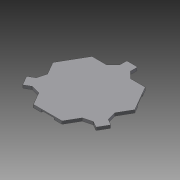
# Autodesk Inventor part: Frame_Bed
Saved by Autodesk Inventor 2014 (Build 180170000, 170)
## iProperties
Created: 2014-08-27
Part Number: Frame_Bed
Material: Generic
Document SubType Name: Modeling
Designer: ThatOtherGuy
Density: 1 g/cm^3
Appearance: Default
Author: ThatOtherGuy
Autodesk Inventor part; units mm, degrees
ref_plane "YZ Plane" through (0, 0, 0) normal (1, 0, 0) x (0, 1, 0)
ref_plane "XZ Plane" through (0, 0, 0) normal (0, 1, 0) x (-1, 0, 0)
ref_plane "XY Plane" through (0, 0, 0) normal (0, 0, 1) x (1, 0, 0)
sketch "Sketch2" plane through (0, 0, 0) normal (0, 0, 1) x (1, 0, 0)
  line L0 (0, 0) -> (-63.75, 36.8061)
  line L1 (63.75, 36.8061) -> (0, 0)
  line L2 (0, 0) -> (147.7389, 0) construction
  line L3 (63.75, 36.8061) -> (42.5, 73.6122)
  line L4 (-42.5, 73.6122) -> (-63.75, 36.8061)
  line L5 (-42.5, 73.6122) -> (42.5, 73.6122)
  line L6 (-12.5, 73.6122) -> (-12.5, 105)
  line L7 (12.5, 105) -> (12.5, 73.6122)
  line L8 (63.75, 36.8061) -> (85, 0) construction
  line L9 (12.5, 88.6122) -> (27.5, 73.6122)
  line L10 (-27.5, 73.6122) -> (-12.5, 88.6122)
  line L11 (63.75, 36.8061) -> (77.9423, 45)
  line L12 (77.9423, 45) -> (61.423, 73.6122)
  line L13 (61.423, 73.6122) -> (42.5, 73.6122)
  line L14 (-63.75, 36.8061) -> (-77.9423, 45)
  line L15 (-77.9423, 45) -> (-61.423, 73.6122)
  line L16 (-61.423, 73.6122) -> (-42.5, 73.6122)
  line L17 (-12.5, 105) -> (12.5, 105)
  dimension "d29" = 120
  dimension "d30" = 30
  dimension "d31" = 30
  dimension "d33" = 25
  dimension "d34" = 85
  dimension "d35" = 60
  dimension "d36" = 85
  dimension "d37" = 45
  dimension "d38" = 15
  dimension "d45" = 90
  dimension "d47" = 105
  constraints: 36 end point, 8 perpendicular, 7 point on line, 5 equal length, 2 collinear, 2 parallel, 1 horizontal
  measures "d29" angle of L0 L1
  measures "d30" angle of L2 L1
  measures "d31" angle of L2 L0
  measures "d33" distance between parallel lines of L6 L7
  measures "d34" distance of L4.start L3.end
  measures "d35" angle of L2 L3
  measures "d36" distance of L8.end L3.end
  measures "d37" angle of L5 L9
  measures "d38" distance of L7.end L9.start
  measures "d45" distance of L11.end L0.start
  measures "d47" distance from line of L0.start L17
extrude "Base" add sketch "Sketch2" along normal blind 6.731
sketch "Sketch3" plane through (0, 0, 0) normal (0, 0, -1) x (-1, 0, 0)
  line L0 (77.9423, 45) -> (0, 0) projected
  line L1 (61.423, 73.6122) -> (77.9423, 45) projected
  line L2 (-77.9423, 45) -> (-61.423, 73.6122) projected
  line L3 (0, 0) -> (-77.9423, 45) projected
  line L4 (-47.6314, 27.5) -> (-40.1314, 40.4904)
  line L5 (-40.1314, 40.4904) -> (-70.4423, 57.9904)
  line L6 (47.6314, 27.5) -> (40.1314, 40.4904)
  line L7 (40.1314, 40.4904) -> (70.4423, 57.9904)
  dimension "d49" = 15
  dimension "d50" = 35
  constraints: 8 end point, 4 point on line, 3 perpendicular, 2 equal length, 1 parallel
  measures "d49" distance between parallel lines of L0 L7
  measures "d50" distance of L6.end L7.end
extrude "CutTabs" cut sketch "Sketch3" against normal blind 4
fillet "Fillet3" radius 1.5875 8 edges at (61.423, 73.6122, 3.3655) (27.5, 73.6122, 3.3655) (12.5, 88.6122, 3.3655) (12.5, 105, 3.3655) (-12.5, 88.6122, 3.3655) (-27.5, 73.6122, 3.3655) (-61.423, 73.6122, 3.3655) (-12.5, 105, 3.3655)
pattern_circular "Circular Pattern1" count 3 over 360 about axis through (0, 0, 0) along (0, 0, 1) of "Base", "Fillet3", "CutTabs"
sketch "DXFExport" plane through (0, 0, 0) normal (0, 0, -1) x (-1, 0, 0)
  arc A0 (-95.8079, -40.8809) -> (-96.3889, -43.0495) centre (-95.0141, -42.2557) ccw projected
  line L0 (-85.4764, -61.9505) -> (-96.3889, -43.0495) projected
  arc A1 (-85.4764, -61.9505) -> (-83.3079, -62.5316) centre (-84.1016, -61.1568) ccw projected
  line L1 (-71.0598, -55.4602) -> (-83.3079, -62.5316) projected
  arc A2 (-69.8552, -55.3016) -> (-71.0598, -55.4602) centre (-70.2661, -56.835) ccw projected
  line L2 (-50.6352, -60.4516) -> (-69.8552, -55.3016) projected
  arc A3 (-49.6712, -61.1912) -> (-50.6352, -60.4516) centre (-51.046, -61.985) ccw projected
  line L3 (-33.4967, -89.2063) -> (-49.6712, -61.1912) projected
  arc A4 (-33.4967, -89.2063) -> (-32.1219, -90) centre (-32.1219, -88.4125) ccw projected
  line L4 (-15, -90) -> (-32.1219, -90) projected
  line L5 (-15, -90) -> (-15, -55) projected
  line L6 (-15, -55) -> (15, -55) projected
  line L7 (15, -55) -> (15, -90) projected
  line L8 (32.1219, -90) -> (15, -90) projected
  arc A5 (32.1219, -90) -> (33.4967, -89.2062) centre (32.1219, -88.4125) ccw projected
  line L9 (49.6712, -61.1912) -> (33.4967, -89.2062) projected
  arc A6 (50.6352, -60.4516) -> (49.6712, -61.1912) centre (51.046, -61.985) ccw projected
  line L10 (69.8552, -55.3016) -> (50.6352, -60.4516) projected
  arc A7 (71.0598, -55.4602) -> (69.8552, -55.3016) centre (70.2661, -56.835) ccw projected
  line L11 (83.3079, -62.5316) -> (71.0598, -55.4602) projected
  arc A8 (83.3079, -62.5316) -> (85.4764, -61.9505) centre (84.1016, -61.1568) ccw projected
  line L12 (96.3889, -43.0495) -> (85.4764, -61.9505) projected
  arc A9 (96.3889, -43.0495) -> (95.8079, -40.8809) centre (95.0141, -42.2557) ccw projected
  line L13 (83.5598, -33.8095) -> (95.8079, -40.8809) projected
  arc A10 (82.8202, -32.8456) -> (83.5598, -33.8095) centre (84.3536, -32.4347) ccw projected
  line L14 (77.6702, -13.6255) -> (82.8202, -32.8456) projected
  arc A11 (77.8288, -12.4209) -> (77.6702, -13.6255) centre (79.2036, -13.2147) ccw projected
  line L15 (94.0033, 15.5941) -> (77.8288, -12.4209) projected
  arc A12 (94.0033, 15.5941) -> (94.0033, 17.1816) centre (92.6284, 16.3878) ccw projected
  line L16 (85.4423, 32.0096) -> (94.0033, 17.1816) projected
  line L17 (85.4423, 32.0096) -> (55.1314, 14.5096) projected
  line L18 (55.1314, 14.5096) -> (40.1314, 40.4904) projected
  line L19 (40.1314, 40.4904) -> (70.4423, 57.9904) projected
  line L20 (61.8813, 72.8184) -> (70.4423, 57.9904) projected
  arc A13 (61.8813, 72.8184) -> (60.5065, 73.6122) centre (60.5065, 72.0247) ccw projected
  line L21 (28.1576, 73.6122) -> (60.5065, 73.6122) projected
  arc A14 (27.035, 74.0771) -> (28.1576, 73.6122) centre (28.1576, 75.1997) ccw projected
  line L22 (12.965, 88.1472) -> (27.035, 74.0771) projected
  arc A15 (12.5, 89.2697) -> (12.965, 88.1472) centre (14.0875, 89.2697) ccw projected
  line L23 (12.5, 103.4125) -> (12.5, 89.2697) projected
  arc A16 (12.5, 103.4125) -> (10.9125, 105) centre (10.9125, 103.4125) ccw projected
  line L24 (-10.9125, 105) -> (10.9125, 105) projected
  arc A17 (-10.9125, 105) -> (-12.5, 103.4125) centre (-10.9125, 103.4125) ccw projected
  line L25 (-12.5, 89.2697) -> (-12.5, 103.4125) projected
  arc A18 (-12.965, 88.1472) -> (-12.5, 89.2697) centre (-14.0875, 89.2697) ccw projected
  line L26 (-27.035, 74.0771) -> (-12.965, 88.1472) projected
  arc A19 (-28.1576, 73.6122) -> (-27.035, 74.0771) centre (-28.1576, 75.1997) ccw projected
  line L27 (-60.5065, 73.6122) -> (-28.1576, 73.6122) projected
  arc A20 (-60.5065, 73.6122) -> (-61.8813, 72.8184) centre (-60.5065, 72.0247) ccw projected
  line L28 (-70.4423, 57.9904) -> (-61.8813, 72.8184) projected
  line L29 (-70.4423, 57.9904) -> (-40.1314, 40.4904) projected
  line L30 (-40.1314, 40.4904) -> (-55.1314, 14.5096) projected
  line L31 (-55.1314, 14.5096) -> (-85.4423, 32.0096) projected
  line L32 (-94.0033, 17.1816) -> (-85.4423, 32.0096) projected
  arc A21 (-94.0033, 17.1816) -> (-94.0033, 15.5941) centre (-92.6284, 16.3878) ccw projected
  line L33 (-77.8288, -12.4209) -> (-94.0033, 15.5941) projected
  arc A22 (-77.6702, -13.6255) -> (-77.8288, -12.4209) centre (-79.2036, -13.2147) ccw projected
  line L34 (-82.8202, -32.8456) -> (-77.6702, -13.6255) projected
  arc A23 (-83.5598, -33.8095) -> (-82.8202, -32.8456) centre (-84.3536, -32.4347) ccw projected
  line L35 (-95.8079, -40.8809) -> (-83.5598, -33.8095) projected
  line L36 (-85.4423, 32.0096) -> (-70.4423, 57.9904)
  line L37 (70.4423, 57.9904) -> (85.4423, 32.0096)
  line L38 (15, -90) -> (-15, -90)
  point P0 (0, 0)
  constraints: 6 end point, 2 perpendicular, 1 parallel
equation "\"d30\" = d31"
equation "\"d36\" = d34"
equation "\"d39\" = THICKB"
equation "\"THICKA\" = 3.175"
equation "\"THICKB\" = 6.731"
equation "\"THICKC\" = 12.7"
equation "\"BALLDIA\" = 12"
equation "\"MAGDIA\" = 9.5"
equation "\"THICKPLY\" = 5"
body "Solid2"
